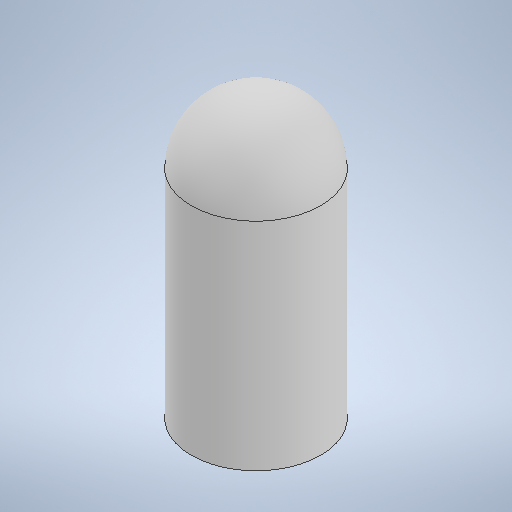
# Autodesk Inventor part: Propane Bottle
Saved by Autodesk Inventor 2025 (Build 290162010, 162A)
## iProperties
Created: 2024-06-12
Part Number: Propane Bottle
Material: Generic
Document SubType Name: Modeling
Designer: Alan Thomas
Mass: 19181.1 g
Surface Area: 4028.31 cm^2
Volume: 19181.1 cm^3
Density: 1 g/cm^3
Appearance: Default
Author: Alan Thomas
Autodesk Inventor part; units mm, degrees
ref_plane "YZ Plane" through (0, 0, 0) normal (1, 0, 0) x (0, 1, 0)
ref_plane "XZ Plane" through (0, 0, 0) normal (0, 1, 0) x (-1, 0, 0)
ref_plane "XY Plane" through (0, 0, 0) normal (0, 0, 1) x (1, 0, 0)
sketch "Sketch1" plane through (0, 0, 0) normal (0, 1, 0) x (-1, 0, 0)
  circle A0 centre (0, 0) radius 115
  dimension "d0" = 230
  constraints: 1 centre point, 1 coincident
  measures "d0" diameter of A0
extrude "Extrusion1" add sketch "Sketch1" along normal blind 500
fillet "Fillet1" radius 115 1 edges at (115, 500, 0)
body "Solid1"
